Autodesk Inventor part; units mm, degrees
(part 3 of 3)
ref_plane "to_Bolt_1_434_YZ" through (140.9639, 0, 300) normal (1, 0, 0) x (0, 0, -1)
ref_plane "to_Bolt_1_434_ZX" through (140.9639, 0, 300) normal (0, 0, -1) x (0, 1, 0)
ref_plane "to_Bolt_1_435_XY" through (143.3735, 0, 300) normal (0, 1, 0) x (1, 0, 0)
ref_plane "to_Bolt_1_435_YZ" through (143.3735, 0, 300) normal (1, 0, 0) x (0, 0, -1)
ref_plane "to_Bolt_1_435_ZX" through (143.3735, 0, 300) normal (0, 0, -1) x (0, 1, 0)
ref_plane "to_Bolt_1_436_XY" through (145.7831, 0, 300) normal (0, 1, 0) x (1, 0, 0)
ref_plane "to_Bolt_1_436_YZ" through (145.7831, 0, 300) normal (1, 0, 0) x (0, 0, -1)
ref_plane "to_Bolt_1_436_ZX" through (145.7831, 0, 300) normal (0, 0, -1) x (0, 1, 0)
ref_plane "to_Bolt_1_437_XY" through (148.1928, 0, 300) normal (0, 1, 0) x (1, 0, 0)
ref_plane "to_Bolt_1_437_YZ" through (148.1928, 0, 300) normal (1, 0, 0) x (0, 0, -1)
ref_plane "to_Bolt_1_437_ZX" through (148.1928, 0, 300) normal (0, 0, -1) x (0, 1, 0)
ref_plane "to_Bolt_1_438_XY" through (150.6024, 0, 300) normal (0, 1, 0) x (1, 0, 0)
ref_plane "to_Bolt_1_438_YZ" through (150.6024, 0, 300) normal (1, 0, 0) x (0, 0, -1)
ref_plane "to_Bolt_1_438_ZX" through (150.6024, 0, 300) normal (0, 0, -1) x (0, 1, 0)
ref_plane "to_Bolt_1_439_XY" through (153.012, 0, 300) normal (0, 1, 0) x (1, 0, 0)
ref_plane "to_Bolt_1_439_YZ" through (153.012, 0, 300) normal (1, 0, 0) x (0, 0, -1)
ref_plane "to_Bolt_1_439_ZX" through (153.012, 0, 300) normal (0, 0, -1) x (0, 1, 0)
ref_plane "to_Bolt_1_44_XY" through (-196.3855, 0, -300) normal (0, 1, 0) x (1, 0, 0)
ref_plane "to_Bolt_1_44_YZ" through (-196.3855, 0, -300) normal (1, 0, 0) x (0, 0, -1)
ref_plane "to_Bolt_1_44_ZX" through (-196.3855, 0, -300) normal (0, 0, -1) x (0, 1, 0)
ref_plane "to_Bolt_1_440_XY" through (155.4217, 0, 300) normal (0, 1, 0) x (1, 0, 0)
ref_plane "to_Bolt_1_440_YZ" through (155.4217, 0, 300) normal (1, 0, 0) x (0, 0, -1)
ref_plane "to_Bolt_1_440_ZX" through (155.4217, 0, 300) normal (0, 0, -1) x (0, 1, 0)
ref_plane "to_Bolt_1_441_XY" through (157.8313, 0, 300) normal (0, 1, 0) x (1, 0, 0)
ref_plane "to_Bolt_1_441_YZ" through (157.8313, 0, 300) normal (1, 0, 0) x (0, 0, -1)
ref_plane "to_Bolt_1_441_ZX" through (157.8313, 0, 300) normal (0, 0, -1) x (0, 1, 0)
ref_plane "to_Bolt_1_442_XY" through (160.241, 0, 300) normal (0, 1, 0) x (1, 0, 0)
ref_plane "to_Bolt_1_442_YZ" through (160.241, 0, 300) normal (1, 0, 0) x (0, 0, -1)
ref_plane "to_Bolt_1_442_ZX" through (160.241, 0, 300) normal (0, 0, -1) x (0, 1, 0)
ref_plane "to_Bolt_1_443_XY" through (162.6506, 0, 300) normal (0, 1, 0) x (1, 0, 0)
ref_plane "to_Bolt_1_443_YZ" through (162.6506, 0, 300) normal (1, 0, 0) x (0, 0, -1)
ref_plane "to_Bolt_1_443_ZX" through (162.6506, 0, 300) normal (0, 0, -1) x (0, 1, 0)
ref_plane "to_Bolt_1_444_XY" through (165.0602, 0, 300) normal (0, 1, 0) x (1, 0, 0)
ref_plane "to_Bolt_1_444_YZ" through (165.0602, 0, 300) normal (1, 0, 0) x (0, 0, -1)
ref_plane "to_Bolt_1_444_ZX" through (165.0602, 0, 300) normal (0, 0, -1) x (0, 1, 0)
ref_plane "to_Bolt_1_445_XY" through (167.4699, 0, 300) normal (0, 1, 0) x (1, 0, 0)
ref_plane "to_Bolt_1_445_YZ" through (167.4699, 0, 300) normal (1, 0, 0) x (0, 0, -1)
ref_plane "to_Bolt_1_445_ZX" through (167.4699, 0, 300) normal (0, 0, -1) x (0, 1, 0)
ref_plane "to_Bolt_1_446_XY" through (169.8795, 0, 300) normal (0, 1, 0) x (1, 0, 0)
ref_plane "to_Bolt_1_446_YZ" through (169.8795, 0, 300) normal (1, 0, 0) x (0, 0, -1)
ref_plane "to_Bolt_1_446_ZX" through (169.8795, 0, 300) normal (0, 0, -1) x (0, 1, 0)
ref_plane "to_Bolt_1_447_XY" through (172.2892, 0, 300) normal (0, 1, 0) x (1, 0, 0)
ref_plane "to_Bolt_1_447_YZ" through (172.2892, 0, 300) normal (1, 0, 0) x (0, 0, -1)
ref_plane "to_Bolt_1_447_ZX" through (172.2892, 0, 300) normal (0, 0, -1) x (0, 1, 0)
ref_plane "to_Bolt_1_448_XY" through (174.6988, 0, 300) normal (0, 1, 0) x (1, 0, 0)
ref_plane "to_Bolt_1_448_YZ" through (174.6988, 0, 300) normal (1, 0, 0) x (0, 0, -1)
ref_plane "to_Bolt_1_448_ZX" through (174.6988, 0, 300) normal (0, 0, -1) x (0, 1, 0)
ref_plane "to_Bolt_1_449_XY" through (177.1084, 0, 300) normal (0, 1, 0) x (1, 0, 0)
ref_plane "to_Bolt_1_449_YZ" through (177.1084, 0, 300) normal (1, 0, 0) x (0, 0, -1)
ref_plane "to_Bolt_1_449_ZX" through (177.1084, 0, 300) normal (0, 0, -1) x (0, 1, 0)
ref_plane "to_Bolt_1_45_XY" through (-193.9759, 0, -300) normal (0, 1, 0) x (1, 0, 0)
ref_plane "to_Bolt_1_45_YZ" through (-193.9759, 0, -300) normal (1, 0, 0) x (0, 0, -1)
ref_plane "to_Bolt_1_45_ZX" through (-193.9759, 0, -300) normal (0, 0, -1) x (0, 1, 0)
ref_plane "to_Bolt_1_450_XY" through (179.5181, 0, 300) normal (0, 1, 0) x (1, 0, 0)
ref_plane "to_Bolt_1_450_YZ" through (179.5181, 0, 300) normal (1, 0, 0) x (0, 0, -1)
ref_plane "to_Bolt_1_450_ZX" through (179.5181, 0, 300) normal (0, 0, -1) x (0, 1, 0)
ref_plane "to_Bolt_1_451_XY" through (181.9277, 0, 300) normal (0, 1, 0) x (1, 0, 0)
ref_plane "to_Bolt_1_451_YZ" through (181.9277, 0, 300) normal (1, 0, 0) x (0, 0, -1)
ref_plane "to_Bolt_1_451_ZX" through (181.9277, 0, 300) normal (0, 0, -1) x (0, 1, 0)
ref_plane "to_Bolt_1_452_XY" through (184.3373, 0, 300) normal (0, 1, 0) x (1, 0, 0)
ref_plane "to_Bolt_1_452_YZ" through (184.3373, 0, 300) normal (1, 0, 0) x (0, 0, -1)
ref_plane "to_Bolt_1_452_ZX" through (184.3373, 0, 300) normal (0, 0, -1) x (0, 1, 0)
ref_plane "to_Bolt_1_453_XY" through (186.747, 0, 300) normal (0, 1, 0) x (1, 0, 0)
ref_plane "to_Bolt_1_453_YZ" through (186.747, 0, 300) normal (1, 0, 0) x (0, 0, -1)
ref_plane "to_Bolt_1_453_ZX" through (186.747, 0, 300) normal (0, 0, -1) x (0, 1, 0)
ref_plane "to_Bolt_1_454_XY" through (189.1566, 0, 300) normal (0, 1, 0) x (1, 0, 0)
ref_plane "to_Bolt_1_454_YZ" through (189.1566, 0, 300) normal (1, 0, 0) x (0, 0, -1)
ref_plane "to_Bolt_1_454_ZX" through (189.1566, 0, 300) normal (0, 0, -1) x (0, 1, 0)
ref_plane "to_Bolt_1_455_XY" through (191.5663, 0, 300) normal (0, 1, 0) x (1, 0, 0)
ref_plane "to_Bolt_1_455_YZ" through (191.5663, 0, 300) normal (1, 0, 0) x (0, 0, -1)
ref_plane "to_Bolt_1_455_ZX" through (191.5663, 0, 300) normal (0, 0, -1) x (0, 1, 0)
ref_plane "to_Bolt_1_456_XY" through (193.9759, 0, 300) normal (0, 1, 0) x (1, 0, 0)
ref_plane "to_Bolt_1_456_YZ" through (193.9759, 0, 300) normal (1, 0, 0) x (0, 0, -1)
ref_plane "to_Bolt_1_456_ZX" through (193.9759, 0, 300) normal (0, 0, -1) x (0, 1, 0)
ref_plane "to_Bolt_1_457_XY" through (196.3855, 0, 300) normal (0, 1, 0) x (1, 0, 0)
ref_plane "to_Bolt_1_457_YZ" through (196.3855, 0, 300) normal (1, 0, 0) x (0, 0, -1)
ref_plane "to_Bolt_1_457_ZX" through (196.3855, 0, 300) normal (0, 0, -1) x (0, 1, 0)
ref_plane "to_Bolt_1_458_XY" through (198.7952, 0, 300) normal (0, 1, 0) x (1, 0, 0)
ref_plane "to_Bolt_1_458_YZ" through (198.7952, 0, 300) normal (1, 0, 0) x (0, 0, -1)
ref_plane "to_Bolt_1_458_ZX" through (198.7952, 0, 300) normal (0, 0, -1) x (0, 1, 0)
ref_plane "to_Bolt_1_459_XY" through (201.2048, 0, 300) normal (0, 1, 0) x (1, 0, 0)
ref_plane "to_Bolt_1_459_YZ" through (201.2048, 0, 300) normal (1, 0, 0) x (0, 0, -1)
ref_plane "to_Bolt_1_459_ZX" through (201.2048, 0, 300) normal (0, 0, -1) x (0, 1, 0)
ref_plane "to_Bolt_1_46_XY" through (-191.5663, 0, -300) normal (0, 1, 0) x (1, 0, 0)
ref_plane "to_Bolt_1_46_YZ" through (-191.5663, 0, -300) normal (1, 0, 0) x (0, 0, -1)
ref_plane "to_Bolt_1_46_ZX" through (-191.5663, 0, -300) normal (0, 0, -1) x (0, 1, 0)
ref_plane "to_Bolt_1_460_XY" through (203.6145, 0, 300) normal (0, 1, 0) x (1, 0, 0)
ref_plane "to_Bolt_1_460_YZ" through (203.6145, 0, 300) normal (1, 0, 0) x (0, 0, -1)
ref_plane "to_Bolt_1_460_ZX" through (203.6145, 0, 300) normal (0, 0, -1) x (0, 1, 0)
ref_plane "to_Bolt_1_461_XY" through (206.0241, 0, 300) normal (0, 1, 0) x (1, 0, 0)
ref_plane "to_Bolt_1_461_YZ" through (206.0241, 0, 300) normal (1, 0, 0) x (0, 0, -1)
ref_plane "to_Bolt_1_461_ZX" through (206.0241, 0, 300) normal (0, 0, -1) x (0, 1, 0)
ref_plane "to_Bolt_1_462_XY" through (208.4337, 0, 300) normal (0, 1, 0) x (1, 0, 0)
ref_plane "to_Bolt_1_462_YZ" through (208.4337, 0, 300) normal (1, 0, 0) x (0, 0, -1)
ref_plane "to_Bolt_1_462_ZX" through (208.4337, 0, 300) normal (0, 0, -1) x (0, 1, 0)
ref_plane "to_Bolt_1_463_XY" through (210.8434, 0, 300) normal (0, 1, 0) x (1, 0, 0)
ref_plane "to_Bolt_1_463_YZ" through (210.8434, 0, 300) normal (1, 0, 0) x (0, 0, -1)
ref_plane "to_Bolt_1_463_ZX" through (210.8434, 0, 300) normal (0, 0, -1) x (0, 1, 0)
ref_plane "to_Bolt_1_464_XY" through (213.253, 0, 300) normal (0, 1, 0) x (1, 0, 0)
ref_plane "to_Bolt_1_464_YZ" through (213.253, 0, 300) normal (1, 0, 0) x (0, 0, -1)
ref_plane "to_Bolt_1_464_ZX" through (213.253, 0, 300) normal (0, 0, -1) x (0, 1, 0)
ref_plane "to_Bolt_1_465_XY" through (215.6627, 0, 300) normal (0, 1, 0) x (1, 0, 0)
ref_plane "to_Bolt_1_465_YZ" through (215.6627, 0, 300) normal (1, 0, 0) x (0, 0, -1)
ref_plane "to_Bolt_1_465_ZX" through (215.6627, 0, 300) normal (0, 0, -1) x (0, 1, 0)
ref_plane "to_Bolt_1_466_XY" through (218.0723, 0, 300) normal (0, 1, 0) x (1, 0, 0)
ref_plane "to_Bolt_1_466_YZ" through (218.0723, 0, 300) normal (1, 0, 0) x (0, 0, -1)
ref_plane "to_Bolt_1_466_ZX" through (218.0723, 0, 300) normal (0, 0, -1) x (0, 1, 0)
ref_plane "to_Bolt_1_467_XY" through (220.4819, 0, 300) normal (0, 1, 0) x (1, 0, 0)
ref_plane "to_Bolt_1_467_YZ" through (220.4819, 0, 300) normal (1, 0, 0) x (0, 0, -1)
ref_plane "to_Bolt_1_467_ZX" through (220.4819, 0, 300) normal (0, 0, -1) x (0, 1, 0)
ref_plane "to_Bolt_1_468_XY" through (222.8916, 0, 300) normal (0, 1, 0) x (1, 0, 0)
ref_plane "to_Bolt_1_468_YZ" through (222.8916, 0, 300) normal (1, 0, 0) x (0, 0, -1)
ref_plane "to_Bolt_1_468_ZX" through (222.8916, 0, 300) normal (0, 0, -1) x (0, 1, 0)
ref_plane "to_Bolt_1_469_XY" through (225.3012, 0, 300) normal (0, 1, 0) x (1, 0, 0)
ref_plane "to_Bolt_1_469_YZ" through (225.3012, 0, 300) normal (1, 0, 0) x (0, 0, -1)
ref_plane "to_Bolt_1_469_ZX" through (225.3012, 0, 300) normal (0, 0, -1) x (0, 1, 0)
ref_plane "to_Bolt_1_47_XY" through (-189.1566, 0, -300) normal (0, 1, 0) x (1, 0, 0)
ref_plane "to_Bolt_1_47_YZ" through (-189.1566, 0, -300) normal (1, 0, 0) x (0, 0, -1)
ref_plane "to_Bolt_1_47_ZX" through (-189.1566, 0, -300) normal (0, 0, -1) x (0, 1, 0)
ref_plane "to_Bolt_1_470_XY" through (227.7108, 0, 300) normal (0, 1, 0) x (1, 0, 0)
ref_plane "to_Bolt_1_470_YZ" through (227.7108, 0, 300) normal (1, 0, 0) x (0, 0, -1)
ref_plane "to_Bolt_1_470_ZX" through (227.7108, 0, 300) normal (0, 0, -1) x (0, 1, 0)
ref_plane "to_Bolt_1_471_XY" through (230.1205, 0, 300) normal (0, 1, 0) x (1, 0, 0)
ref_plane "to_Bolt_1_471_YZ" through (230.1205, 0, 300) normal (1, 0, 0) x (0, 0, -1)
ref_plane "to_Bolt_1_471_ZX" through (230.1205, 0, 300) normal (0, 0, -1) x (0, 1, 0)
ref_plane "to_Bolt_1_472_XY" through (232.5301, 0, 300) normal (0, 1, 0) x (1, 0, 0)
ref_plane "to_Bolt_1_472_YZ" through (232.5301, 0, 300) normal (1, 0, 0) x (0, 0, -1)
ref_plane "to_Bolt_1_472_ZX" through (232.5301, 0, 300) normal (0, 0, -1) x (0, 1, 0)
ref_plane "to_Bolt_1_473_XY" through (234.9398, 0, 300) normal (0, 1, 0) x (1, 0, 0)
ref_plane "to_Bolt_1_473_YZ" through (234.9398, 0, 300) normal (1, 0, 0) x (0, 0, -1)
ref_plane "to_Bolt_1_473_ZX" through (234.9398, 0, 300) normal (0, 0, -1) x (0, 1, 0)
ref_plane "to_Bolt_1_474_XY" through (237.3494, 0, 300) normal (0, 1, 0) x (1, 0, 0)
ref_plane "to_Bolt_1_474_YZ" through (237.3494, 0, 300) normal (1, 0, 0) x (0, 0, -1)
ref_plane "to_Bolt_1_474_ZX" through (237.3494, 0, 300) normal (0, 0, -1) x (0, 1, 0)
ref_plane "to_Bolt_1_475_XY" through (239.759, 0, 300) normal (0, 1, 0) x (1, 0, 0)
ref_plane "to_Bolt_1_475_YZ" through (239.759, 0, 300) normal (1, 0, 0) x (0, 0, -1)
ref_plane "to_Bolt_1_475_ZX" through (239.759, 0, 300) normal (0, 0, -1) x (0, 1, 0)
ref_plane "to_Bolt_1_476_XY" through (242.1687, 0, 300) normal (0, 1, 0) x (1, 0, 0)
ref_plane "to_Bolt_1_476_YZ" through (242.1687, 0, 300) normal (1, 0, 0) x (0, 0, -1)
ref_plane "to_Bolt_1_476_ZX" through (242.1687, 0, 300) normal (0, 0, -1) x (0, 1, 0)
ref_plane "to_Bolt_1_477_XY" through (244.5783, 0, 300) normal (0, 1, 0) x (1, 0, 0)
ref_plane "to_Bolt_1_477_YZ" through (244.5783, 0, 300) normal (1, 0, 0) x (0, 0, -1)
ref_plane "to_Bolt_1_477_ZX" through (244.5783, 0, 300) normal (0, 0, -1) x (0, 1, 0)
ref_plane "to_Bolt_1_478_XY" through (246.988, 0, 300) normal (0, 1, 0) x (1, 0, 0)
ref_plane "to_Bolt_1_478_YZ" through (246.988, 0, 300) normal (1, 0, 0) x (0, 0, -1)
ref_plane "to_Bolt_1_478_ZX" through (246.988, 0, 300) normal (0, 0, -1) x (0, 1, 0)
ref_plane "to_Bolt_1_479_XY" through (249.3976, 0, 300) normal (0, 1, 0) x (1, 0, 0)
ref_plane "to_Bolt_1_479_YZ" through (249.3976, 0, 300) normal (1, 0, 0) x (0, 0, -1)
ref_plane "to_Bolt_1_479_ZX" through (249.3976, 0, 300) normal (0, 0, -1) x (0, 1, 0)
ref_plane "to_Bolt_1_48_XY" through (-186.747, 0, -300) normal (0, 1, 0) x (1, 0, 0)
ref_plane "to_Bolt_1_48_YZ" through (-186.747, 0, -300) normal (1, 0, 0) x (0, 0, -1)
ref_plane "to_Bolt_1_48_ZX" through (-186.747, 0, -300) normal (0, 0, -1) x (0, 1, 0)
ref_plane "to_Bolt_1_480_XY" through (251.8072, 0, 300) normal (0, 1, 0) x (1, 0, 0)
ref_plane "to_Bolt_1_480_YZ" through (251.8072, 0, 300) normal (1, 0, 0) x (0, 0, -1)
ref_plane "to_Bolt_1_480_ZX" through (251.8072, 0, 300) normal (0, 0, -1) x (0, 1, 0)
ref_plane "to_Bolt_1_481_XY" through (254.2169, 0, 300) normal (0, 1, 0) x (1, 0, 0)
ref_plane "to_Bolt_1_481_YZ" through (254.2169, 0, 300) normal (1, 0, 0) x (0, 0, -1)
ref_plane "to_Bolt_1_481_ZX" through (254.2169, 0, 300) normal (0, 0, -1) x (0, 1, 0)
ref_plane "to_Bolt_1_482_XY" through (256.6265, 0, 300) normal (0, 1, 0) x (1, 0, 0)
ref_plane "to_Bolt_1_482_YZ" through (256.6265, 0, 300) normal (1, 0, 0) x (0, 0, -1)
ref_plane "to_Bolt_1_482_ZX" through (256.6265, 0, 300) normal (0, 0, -1) x (0, 1, 0)
ref_plane "to_Bolt_1_483_XY" through (259.0361, 0, 300) normal (0, 1, 0) x (1, 0, 0)
ref_plane "to_Bolt_1_483_YZ" through (259.0361, 0, 300) normal (1, 0, 0) x (0, 0, -1)
ref_plane "to_Bolt_1_483_ZX" through (259.0361, 0, 300) normal (0, 0, -1) x (0, 1, 0)
ref_plane "to_Bolt_1_484_XY" through (261.4458, 0, 300) normal (0, 1, 0) x (1, 0, 0)
ref_plane "to_Bolt_1_484_YZ" through (261.4458, 0, 300) normal (1, 0, 0) x (0, 0, -1)
ref_plane "to_Bolt_1_484_ZX" through (261.4458, 0, 300) normal (0, 0, -1) x (0, 1, 0)
ref_plane "to_Bolt_1_485_XY" through (263.8554, 0, 300) normal (0, 1, 0) x (1, 0, 0)
ref_plane "to_Bolt_1_485_YZ" through (263.8554, 0, 300) normal (1, 0, 0) x (0, 0, -1)
ref_plane "to_Bolt_1_485_ZX" through (263.8554, 0, 300) normal (0, 0, -1) x (0, 1, 0)
ref_plane "to_Bolt_1_486_XY" through (266.2651, 0, 300) normal (0, 1, 0) x (1, 0, 0)
ref_plane "to_Bolt_1_486_YZ" through (266.2651, 0, 300) normal (1, 0, 0) x (0, 0, -1)
ref_plane "to_Bolt_1_486_ZX" through (266.2651, 0, 300) normal (0, 0, -1) x (0, 1, 0)
ref_plane "to_Bolt_1_487_XY" through (268.6747, 0, 300) normal (0, 1, 0) x (1, 0, 0)
ref_plane "to_Bolt_1_487_YZ" through (268.6747, 0, 300) normal (1, 0, 0) x (0, 0, -1)
ref_plane "to_Bolt_1_487_ZX" through (268.6747, 0, 300) normal (0, 0, -1) x (0, 1, 0)
ref_plane "to_Bolt_1_488_XY" through (271.0843, 0, 300) normal (0, 1, 0) x (1, 0, 0)
ref_plane "to_Bolt_1_488_YZ" through (271.0843, 0, 300) normal (1, 0, 0) x (0, 0, -1)
ref_plane "to_Bolt_1_488_ZX" through (271.0843, 0, 300) normal (0, 0, -1) x (0, 1, 0)
ref_plane "to_Bolt_1_489_XY" through (273.494, 0, 300) normal (0, 1, 0) x (1, 0, 0)
ref_plane "to_Bolt_1_489_YZ" through (273.494, 0, 300) normal (1, 0, 0) x (0, 0, -1)
ref_plane "to_Bolt_1_489_ZX" through (273.494, 0, 300) normal (0, 0, -1) x (0, 1, 0)
ref_plane "to_Bolt_1_49_XY" through (-184.3373, 0, -300) normal (0, 1, 0) x (1, 0, 0)
ref_plane "to_Bolt_1_49_YZ" through (-184.3373, 0, -300) normal (1, 0, 0) x (0, 0, -1)
ref_plane "to_Bolt_1_49_ZX" through (-184.3373, 0, -300) normal (0, 0, -1) x (0, 1, 0)
ref_plane "to_Bolt_1_490_XY" through (275.9036, 0, 300) normal (0, 1, 0) x (1, 0, 0)
ref_plane "to_Bolt_1_490_YZ" through (275.9036, 0, 300) normal (1, 0, 0) x (0, 0, -1)
ref_plane "to_Bolt_1_490_ZX" through (275.9036, 0, 300) normal (0, 0, -1) x (0, 1, 0)
ref_plane "to_Bolt_1_491_XY" through (278.3133, 0, 300) normal (0, 1, 0) x (1, 0, 0)
ref_plane "to_Bolt_1_491_YZ" through (278.3133, 0, 300) normal (1, 0, 0) x (0, 0, -1)
ref_plane "to_Bolt_1_491_ZX" through (278.3133, 0, 300) normal (0, 0, -1) x (0, 1, 0)
ref_plane "to_Bolt_1_492_XY" through (280.7229, 0, 300) normal (0, 1, 0) x (1, 0, 0)
ref_plane "to_Bolt_1_492_YZ" through (280.7229, 0, 300) normal (1, 0, 0) x (0, 0, -1)
ref_plane "to_Bolt_1_492_ZX" through (280.7229, 0, 300) normal (0, 0, -1) x (0, 1, 0)
ref_plane "to_Bolt_1_493_XY" through (283.1325, 0, 300) normal (0, 1, 0) x (1, 0, 0)
ref_plane "to_Bolt_1_493_YZ" through (283.1325, 0, 300) normal (1, 0, 0) x (0, 0, -1)
ref_plane "to_Bolt_1_493_ZX" through (283.1325, 0, 300) normal (0, 0, -1) x (0, 1, 0)
ref_plane "to_Bolt_1_494_XY" through (285.5422, 0, 300) normal (0, 1, 0) x (1, 0, 0)
ref_plane "to_Bolt_1_494_YZ" through (285.5422, 0, 300) normal (1, 0, 0) x (0, 0, -1)
ref_plane "to_Bolt_1_494_ZX" through (285.5422, 0, 300) normal (0, 0, -1) x (0, 1, 0)
ref_plane "to_Bolt_1_495_XY" through (287.9518, 0, 300) normal (0, 1, 0) x (1, 0, 0)
ref_plane "to_Bolt_1_495_YZ" through (287.9518, 0, 300) normal (1, 0, 0) x (0, 0, -1)
ref_plane "to_Bolt_1_495_ZX" through (287.9518, 0, 300) normal (0, 0, -1) x (0, 1, 0)
ref_plane "to_Bolt_1_496_XY" through (290.3614, 0, 300) normal (0, 1, 0) x (1, 0, 0)
ref_plane "to_Bolt_1_496_YZ" through (290.3614, 0, 300) normal (1, 0, 0) x (0, 0, -1)
ref_plane "to_Bolt_1_496_ZX" through (290.3614, 0, 300) normal (0, 0, -1) x (0, 1, 0)
ref_plane "to_Bolt_1_497_XY" through (292.7711, 0, 300) normal (0, 1, 0) x (1, 0, 0)
ref_plane "to_Bolt_1_497_YZ" through (292.7711, 0, 300) normal (1, 0, 0) x (0, 0, -1)
ref_plane "to_Bolt_1_497_ZX" through (292.7711, 0, 300) normal (0, 0, -1) x (0, 1, 0)
ref_plane "to_Bolt_1_498_XY" through (295.1807, 0, 300) normal (0, 1, 0) x (1, 0, 0)
ref_plane "to_Bolt_1_498_YZ" through (295.1807, 0, 300) normal (1, 0, 0) x (0, 0, -1)
ref_plane "to_Bolt_1_498_ZX" through (295.1807, 0, 300) normal (0, 0, -1) x (0, 1, 0)
ref_plane "to_Bolt_1_499_XY" through (297.5904, 0, 300) normal (0, 1, 0) x (1, 0, 0)
ref_plane "to_Bolt_1_499_YZ" through (297.5904, 0, 300) normal (1, 0, 0) x (0, 0, -1)
ref_plane "to_Bolt_1_499_ZX" through (297.5904, 0, 300) normal (0, 0, -1) x (0, 1, 0)
ref_plane "to_Bolt_1_5_XY" through (-290.3614, 0, -300) normal (0, 1, 0) x (1, 0, 0)
ref_plane "to_Bolt_1_5_YZ" through (-290.3614, 0, -300) normal (1, 0, 0) x (0, 0, -1)
ref_plane "to_Bolt_1_5_ZX" through (-290.3614, 0, -300) normal (0, 0, -1) x (0, 1, 0)
ref_plane "to_Bolt_1_50_XY" through (-181.9277, 0, -300) normal (0, 1, 0) x (1, 0, 0)
ref_plane "to_Bolt_1_50_YZ" through (-181.9277, 0, -300) normal (1, 0, 0) x (0, 0, -1)
ref_plane "to_Bolt_1_50_ZX" through (-181.9277, 0, -300) normal (0, 0, -1) x (0, 1, 0)
ref_plane "to_Bolt_1_500_XY" through (300, 0, 300) normal (0, 1, 0) x (1, 0, 0)
ref_plane "to_Bolt_1_500_YZ" through (300, 0, 300) normal (1, 0, 0) x (0, 0, -1)
ref_plane "to_Bolt_1_500_ZX" through (300, 0, 300) normal (0, 0, -1) x (0, 1, 0)
ref_plane "to_Bolt_1_51_XY" through (-179.5181, 0, -300) normal (0, 1, 0) x (1, 0, 0)
ref_plane "to_Bolt_1_51_YZ" through (-179.5181, 0, -300) normal (1, 0, 0) x (0, 0, -1)
ref_plane "to_Bolt_1_51_ZX" through (-179.5181, 0, -300) normal (0, 0, -1) x (0, 1, 0)
ref_plane "to_Bolt_1_52_XY" through (-177.1084, 0, -300) normal (0, 1, 0) x (1, 0, 0)
ref_plane "to_Bolt_1_52_YZ" through (-177.1084, 0, -300) normal (1, 0, 0) x (0, 0, -1)
ref_plane "to_Bolt_1_52_ZX" through (-177.1084, 0, -300) normal (0, 0, -1) x (0, 1, 0)
ref_plane "to_Bolt_1_53_XY" through (-174.6988, 0, -300) normal (0, 1, 0) x (1, 0, 0)
ref_plane "to_Bolt_1_53_YZ" through (-174.6988, 0, -300) normal (1, 0, 0) x (0, 0, -1)
ref_plane "to_Bolt_1_53_ZX" through (-174.6988, 0, -300) normal (0, 0, -1) x (0, 1, 0)
ref_plane "to_Bolt_1_54_XY" through (-172.2892, 0, -300) normal (0, 1, 0) x (1, 0, 0)
ref_plane "to_Bolt_1_54_YZ" through (-172.2892, 0, -300) normal (1, 0, 0) x (0, 0, -1)
ref_plane "to_Bolt_1_54_ZX" through (-172.2892, 0, -300) normal (0, 0, -1) x (0, 1, 0)
ref_plane "to_Bolt_1_55_XY" through (-169.8795, 0, -300) normal (0, 1, 0) x (1, 0, 0)
ref_plane "to_Bolt_1_55_YZ" through (-169.8795, 0, -300) normal (1, 0, 0) x (0, 0, -1)
ref_plane "to_Bolt_1_55_ZX" through (-169.8795, 0, -300) normal (0, 0, -1) x (0, 1, 0)
ref_plane "to_Bolt_1_56_XY" through (-167.4699, 0, -300) normal (0, 1, 0) x (1, 0, 0)
ref_plane "to_Bolt_1_56_YZ" through (-167.4699, 0, -300) normal (1, 0, 0) x (0, 0, -1)
ref_plane "to_Bolt_1_56_ZX" through (-167.4699, 0, -300) normal (0, 0, -1) x (0, 1, 0)
ref_plane "to_Bolt_1_57_XY" through (-165.0602, 0, -300) normal (0, 1, 0) x (1, 0, 0)
ref_plane "to_Bolt_1_57_YZ" through (-165.0602, 0, -300) normal (1, 0, 0) x (0, 0, -1)
ref_plane "to_Bolt_1_57_ZX" through (-165.0602, 0, -300) normal (0, 0, -1) x (0, 1, 0)
ref_plane "to_Bolt_1_58_XY" through (-162.6506, 0, -300) normal (0, 1, 0) x (1, 0, 0)
ref_plane "to_Bolt_1_58_YZ" through (-162.6506, 0, -300) normal (1, 0, 0) x (0, 0, -1)
ref_plane "to_Bolt_1_58_ZX" through (-162.6506, 0, -300) normal (0, 0, -1) x (0, 1, 0)
ref_plane "to_Bolt_1_59_XY" through (-160.241, 0, -300) normal (0, 1, 0) x (1, 0, 0)
ref_plane "to_Bolt_1_59_YZ" through (-160.241, 0, -300) normal (1, 0, 0) x (0, 0, -1)
ref_plane "to_Bolt_1_59_ZX" through (-160.241, 0, -300) normal (0, 0, -1) x (0, 1, 0)
ref_plane "to_Bolt_1_6_XY" through (-287.9518, 0, -300) normal (0, 1, 0) x (1, 0, 0)
ref_plane "to_Bolt_1_6_YZ" through (-287.9518, 0, -300) normal (1, 0, 0) x (0, 0, -1)
ref_plane "to_Bolt_1_6_ZX" through (-287.9518, 0, -300) normal (0, 0, -1) x (0, 1, 0)
ref_plane "to_Bolt_1_60_XY" through (-157.8313, 0, -300) normal (0, 1, 0) x (1, 0, 0)
ref_plane "to_Bolt_1_60_YZ" through (-157.8313, 0, -300) normal (1, 0, 0) x (0, 0, -1)
ref_plane "to_Bolt_1_60_ZX" through (-157.8313, 0, -300) normal (0, 0, -1) x (0, 1, 0)
ref_plane "to_Bolt_1_61_XY" through (-155.4217, 0, -300) normal (0, 1, 0) x (1, 0, 0)
ref_plane "to_Bolt_1_61_YZ" through (-155.4217, 0, -300) normal (1, 0, 0) x (0, 0, -1)
ref_plane "to_Bolt_1_61_ZX" through (-155.4217, 0, -300) normal (0, 0, -1) x (0, 1, 0)
ref_plane "to_Bolt_1_62_XY" through (-153.012, 0, -300) normal (0, 1, 0) x (1, 0, 0)
ref_plane "to_Bolt_1_62_YZ" through (-153.012, 0, -300) normal (1, 0, 0) x (0, 0, -1)
ref_plane "to_Bolt_1_62_ZX" through (-153.012, 0, -300) normal (0, 0, -1) x (0, 1, 0)
ref_plane "to_Bolt_1_63_XY" through (-150.6024, 0, -300) normal (0, 1, 0) x (1, 0, 0)
ref_plane "to_Bolt_1_63_YZ" through (-150.6024, 0, -300) normal (1, 0, 0) x (0, 0, -1)
ref_plane "to_Bolt_1_63_ZX" through (-150.6024, 0, -300) normal (0, 0, -1) x (0, 1, 0)
ref_plane "to_Bolt_1_64_XY" through (-148.1928, 0, -300) normal (0, 1, 0) x (1, 0, 0)
ref_plane "to_Bolt_1_64_YZ" through (-148.1928, 0, -300) normal (1, 0, 0) x (0, 0, -1)
ref_plane "to_Bolt_1_64_ZX" through (-148.1928, 0, -300) normal (0, 0, -1) x (0, 1, 0)
ref_plane "to_Bolt_1_65_XY" through (-145.7831, 0, -300) normal (0, 1, 0) x (1, 0, 0)
ref_plane "to_Bolt_1_65_YZ" through (-145.7831, 0, -300) normal (1, 0, 0) x (0, 0, -1)
ref_plane "to_Bolt_1_65_ZX" through (-145.7831, 0, -300) normal (0, 0, -1) x (0, 1, 0)
ref_plane "to_Bolt_1_66_XY" through (-143.3735, 0, -300) normal (0, 1, 0) x (1, 0, 0)
ref_plane "to_Bolt_1_66_YZ" through (-143.3735, 0, -300) normal (1, 0, 0) x (0, 0, -1)
ref_plane "to_Bolt_1_66_ZX" through (-143.3735, 0, -300) normal (0, 0, -1) x (0, 1, 0)
ref_plane "to_Bolt_1_67_XY" through (-140.9639, 0, -300) normal (0, 1, 0) x (1, 0, 0)
ref_plane "to_Bolt_1_67_YZ" through (-140.9639, 0, -300) normal (1, 0, 0) x (0, 0, -1)
ref_plane "to_Bolt_1_67_ZX" through (-140.9639, 0, -300) normal (0, 0, -1) x (0, 1, 0)
ref_plane "to_Bolt_1_68_XY" through (-138.5542, 0, -300) normal (0, 1, 0) x (1, 0, 0)
ref_plane "to_Bolt_1_68_YZ" through (-138.5542, 0, -300) normal (1, 0, 0) x (0, 0, -1)
ref_plane "to_Bolt_1_68_ZX" through (-138.5542, 0, -300) normal (0, 0, -1) x (0, 1, 0)
ref_plane "to_Bolt_1_69_XY" through (-136.1446, 0, -300) normal (0, 1, 0) x (1, 0, 0)
ref_plane "to_Bolt_1_69_YZ" through (-136.1446, 0, -300) normal (1, 0, 0) x (0, 0, -1)
ref_plane "to_Bolt_1_69_ZX" through (-136.1446, 0, -300) normal (0, 0, -1) x (0, 1, 0)
ref_plane "to_Bolt_1_7_XY" through (-285.5422, 0, -300) normal (0, 1, 0) x (1, 0, 0)
ref_plane "to_Bolt_1_7_YZ" through (-285.5422, 0, -300) normal (1, 0, 0) x (0, 0, -1)
ref_plane "to_Bolt_1_7_ZX" through (-285.5422, 0, -300) normal (0, 0, -1) x (0, 1, 0)
ref_plane "to_Bolt_1_70_XY" through (-133.7349, 0, -300) normal (0, 1, 0) x (1, 0, 0)
ref_plane "to_Bolt_1_70_YZ" through (-133.7349, 0, -300) normal (1, 0, 0) x (0, 0, -1)
ref_plane "to_Bolt_1_70_ZX" through (-133.7349, 0, -300) normal (0, 0, -1) x (0, 1, 0)
ref_plane "to_Bolt_1_71_XY" through (-131.3253, 0, -300) normal (0, 1, 0) x (1, 0, 0)
ref_plane "to_Bolt_1_71_YZ" through (-131.3253, 0, -300) normal (1, 0, 0) x (0, 0, -1)
ref_plane "to_Bolt_1_71_ZX" through (-131.3253, 0, -300) normal (0, 0, -1) x (0, 1, 0)
ref_plane "to_Bolt_1_72_XY" through (-128.9157, 0, -300) normal (0, 1, 0) x (1, 0, 0)
ref_plane "to_Bolt_1_72_YZ" through (-128.9157, 0, -300) normal (1, 0, 0) x (0, 0, -1)
ref_plane "to_Bolt_1_72_ZX" through (-128.9157, 0, -300) normal (0, 0, -1) x (0, 1, 0)
ref_plane "to_Bolt_1_73_XY" through (-126.506, 0, -300) normal (0, 1, 0) x (1, 0, 0)
ref_plane "to_Bolt_1_73_YZ" through (-126.506, 0, -300) normal (1, 0, 0) x (0, 0, -1)
ref_plane "to_Bolt_1_73_ZX" through (-126.506, 0, -300) normal (0, 0, -1) x (0, 1, 0)
ref_plane "to_Bolt_1_74_XY" through (-124.0964, 0, -300) normal (0, 1, 0) x (1, 0, 0)
ref_plane "to_Bolt_1_74_YZ" through (-124.0964, 0, -300) normal (1, 0, 0) x (0, 0, -1)
ref_plane "to_Bolt_1_74_ZX" through (-124.0964, 0, -300) normal (0, 0, -1) x (0, 1, 0)
ref_plane "to_Bolt_1_75_XY" through (-121.6867, 0, -300) normal (0, 1, 0) x (1, 0, 0)
ref_plane "to_Bolt_1_75_YZ" through (-121.6867, 0, -300) normal (1, 0, 0) x (0, 0, -1)
ref_plane "to_Bolt_1_75_ZX" through (-121.6867, 0, -300) normal (0, 0, -1) x (0, 1, 0)
ref_plane "to_Bolt_1_76_XY" through (-119.2771, 0, -300) normal (0, 1, 0) x (1, 0, 0)
ref_plane "to_Bolt_1_76_YZ" through (-119.2771, 0, -300) normal (1, 0, 0) x (0, 0, -1)
ref_plane "to_Bolt_1_76_ZX" through (-119.2771, 0, -300) normal (0, 0, -1) x (0, 1, 0)
ref_plane "to_Bolt_1_77_XY" through (-116.8675, 0, -300) normal (0, 1, 0) x (1, 0, 0)
ref_plane "to_Bolt_1_77_YZ" through (-116.8675, 0, -300) normal (1, 0, 0) x (0, 0, -1)
ref_plane "to_Bolt_1_77_ZX" through (-116.8675, 0, -300) normal (0, 0, -1) x (0, 1, 0)
ref_plane "to_Bolt_1_78_XY" through (-114.4578, 0, -300) normal (0, 1, 0) x (1, 0, 0)
ref_plane "to_Bolt_1_78_YZ" through (-114.4578, 0, -300) normal (1, 0, 0) x (0, 0, -1)
ref_plane "to_Bolt_1_78_ZX" through (-114.4578, 0, -300) normal (0, 0, -1) x (0, 1, 0)
ref_plane "to_Bolt_1_79_XY" through (-112.0482, 0, -300) normal (0, 1, 0) x (1, 0, 0)
ref_plane "to_Bolt_1_79_YZ" through (-112.0482, 0, -300) normal (1, 0, 0) x (0, 0, -1)
ref_plane "to_Bolt_1_79_ZX" through (-112.0482, 0, -300) normal (0, 0, -1) x (0, 1, 0)
ref_plane "to_Bolt_1_8_XY" through (-283.1325, 0, -300) normal (0, 1, 0) x (1, 0, 0)
ref_plane "to_Bolt_1_8_YZ" through (-283.1325, 0, -300) normal (1, 0, 0) x (0, 0, -1)
ref_plane "to_Bolt_1_8_ZX" through (-283.1325, 0, -300) normal (0, 0, -1) x (0, 1, 0)
ref_plane "to_Bolt_1_80_XY" through (-109.6386, 0, -300) normal (0, 1, 0) x (1, 0, 0)
ref_plane "to_Bolt_1_80_YZ" through (-109.6386, 0, -300) normal (1, 0, 0) x (0, 0, -1)
ref_plane "to_Bolt_1_80_ZX" through (-109.6386, 0, -300) normal (0, 0, -1) x (0, 1, 0)
ref_plane "to_Bolt_1_81_XY" through (-107.2289, 0, -300) normal (0, 1, 0) x (1, 0, 0)
ref_plane "to_Bolt_1_81_YZ" through (-107.2289, 0, -300) normal (1, 0, 0) x (0, 0, -1)
ref_plane "to_Bolt_1_81_ZX" through (-107.2289, 0, -300) normal (0, 0, -1) x (0, 1, 0)
ref_plane "to_Bolt_1_82_XY" through (-104.8193, 0, -300) normal (0, 1, 0) x (1, 0, 0)
ref_plane "to_Bolt_1_82_YZ" through (-104.8193, 0, -300) normal (1, 0, 0) x (0, 0, -1)
ref_plane "to_Bolt_1_82_ZX" through (-104.8193, 0, -300) normal (0, 0, -1) x (0, 1, 0)
ref_plane "to_Bolt_1_83_XY" through (-102.4096, 0, -300) normal (0, 1, 0) x (1, 0, 0)
ref_plane "to_Bolt_1_83_YZ" through (-102.4096, 0, -300) normal (1, 0, 0) x (0, 0, -1)
ref_plane "to_Bolt_1_83_ZX" through (-102.4096, 0, -300) normal (0, 0, -1) x (0, 1, 0)
ref_plane "to_Bolt_1_84_XY" through (-100, 0, -300) normal (0, 1, 0) x (1, 0, 0)
ref_plane "to_Bolt_1_84_YZ" through (-100, 0, -300) normal (1, 0, 0) x (0, 0, -1)
ref_plane "to_Bolt_1_84_ZX" through (-100, 0, -300) normal (0, 0, -1) x (0, 1, 0)
ref_plane "to_Bolt_1_85_XY" through (-97.5904, 0, -300) normal (0, 1, 0) x (1, 0, 0)
ref_plane "to_Bolt_1_85_YZ" through (-97.5904, 0, -300) normal (1, 0, 0) x (0, 0, -1)
ref_plane "to_Bolt_1_85_ZX" through (-97.5904, 0, -300) normal (0, 0, -1) x (0, 1, 0)
ref_plane "to_Bolt_1_86_XY" through (-95.1807, 0, -300) normal (0, 1, 0) x (1, 0, 0)
ref_plane "to_Bolt_1_86_YZ" through (-95.1807, 0, -300) normal (1, 0, 0) x (0, 0, -1)
ref_plane "to_Bolt_1_86_ZX" through (-95.1807, 0, -300) normal (0, 0, -1) x (0, 1, 0)
ref_plane "to_Bolt_1_87_XY" through (-92.7711, 0, -300) normal (0, 1, 0) x (1, 0, 0)
ref_plane "to_Bolt_1_87_YZ" through (-92.7711, 0, -300) normal (1, 0, 0) x (0, 0, -1)
ref_plane "to_Bolt_1_87_ZX" through (-92.7711, 0, -300) normal (0, 0, -1) x (0, 1, 0)
ref_plane "to_Bolt_1_88_XY" through (-90.3614, 0, -300) normal (0, 1, 0) x (1, 0, 0)
ref_plane "to_Bolt_1_88_YZ" through (-90.3614, 0, -300) normal (1, 0, 0) x (0, 0, -1)
ref_plane "to_Bolt_1_88_ZX" through (-90.3614, 0, -300) normal (0, 0, -1) x (0, 1, 0)
ref_plane "to_Bolt_1_89_XY" through (-87.9518, 0, -300) normal (0, 1, 0) x (1, 0, 0)
ref_plane "to_Bolt_1_89_YZ" through (-87.9518, 0, -300) normal (1, 0, 0) x (0, 0, -1)
ref_plane "to_Bolt_1_89_ZX" through (-87.9518, 0, -300) normal (0, 0, -1) x (0, 1, 0)
ref_plane "to_Bolt_1_9_XY" through (-280.7229, 0, -300) normal (0, 1, 0) x (1, 0, 0)
ref_plane "to_Bolt_1_9_YZ" through (-280.7229, 0, -300) normal (1, 0, 0) x (0, 0, -1)
ref_plane "to_Bolt_1_9_ZX" through (-280.7229, 0, -300) normal (0, 0, -1) x (0, 1, 0)
ref_plane "to_Bolt_1_90_XY" through (-85.5422, 0, -300) normal (0, 1, 0) x (1, 0, 0)
ref_plane "to_Bolt_1_90_YZ" through (-85.5422, 0, -300) normal (1, 0, 0) x (0, 0, -1)
ref_plane "to_Bolt_1_90_ZX" through (-85.5422, 0, -300) normal (0, 0, -1) x (0, 1, 0)
ref_plane "to_Bolt_1_91_XY" through (-83.1325, 0, -300) normal (0, 1, 0) x (1, 0, 0)
ref_plane "to_Bolt_1_91_YZ" through (-83.1325, 0, -300) normal (1, 0, 0) x (0, 0, -1)
ref_plane "to_Bolt_1_91_ZX" through (-83.1325, 0, -300) normal (0, 0, -1) x (0, 1, 0)
ref_plane "to_Bolt_1_92_XY" through (-80.7229, 0, -300) normal (0, 1, 0) x (1, 0, 0)
ref_plane "to_Bolt_1_92_YZ" through (-80.7229, 0, -300) normal (1, 0, 0) x (0, 0, -1)
ref_plane "to_Bolt_1_92_ZX" through (-80.7229, 0, -300) normal (0, 0, -1) x (0, 1, 0)
ref_plane "to_Bolt_1_93_XY" through (-78.3133, 0, -300) normal (0, 1, 0) x (1, 0, 0)
ref_plane "to_Bolt_1_93_YZ" through (-78.3133, 0, -300) normal (1, 0, 0) x (0, 0, -1)
ref_plane "to_Bolt_1_93_ZX" through (-78.3133, 0, -300) normal (0, 0, -1) x (0, 1, 0)
ref_plane "to_Bolt_1_94_XY" through (-75.9036, 0, -300) normal (0, 1, 0) x (1, 0, 0)
ref_plane "to_Bolt_1_94_YZ" through (-75.9036, 0, -300) normal (1, 0, 0) x (0, 0, -1)
ref_plane "to_Bolt_1_94_ZX" through (-75.9036, 0, -300) normal (0, 0, -1) x (0, 1, 0)
ref_plane "to_Bolt_1_95_XY" through (-73.494, 0, -300) normal (0, 1, 0) x (1, 0, 0)
ref_plane "to_Bolt_1_95_YZ" through (-73.494, 0, -300) normal (1, 0, 0) x (0, 0, -1)
ref_plane "to_Bolt_1_95_ZX" through (-73.494, 0, -300) normal (0, 0, -1) x (0, 1, 0)
ref_plane "to_Bolt_1_96_XY" through (-71.0843, 0, -300) normal (0, 1, 0) x (1, 0, 0)
ref_plane "to_Bolt_1_96_YZ" through (-71.0843, 0, -300) normal (1, 0, 0) x (0, 0, -1)
ref_plane "to_Bolt_1_96_ZX" through (-71.0843, 0, -300) normal (0, 0, -1) x (0, 1, 0)
ref_plane "to_Bolt_1_97_XY" through (-68.6747, 0, -300) normal (0, 1, 0) x (1, 0, 0)
ref_plane "to_Bolt_1_97_YZ" through (-68.6747, 0, -300) normal (1, 0, 0) x (0, 0, -1)
ref_plane "to_Bolt_1_97_ZX" through (-68.6747, 0, -300) normal (0, 0, -1) x (0, 1, 0)
ref_plane "to_Bolt_1_98_XY" through (-66.2651, 0, -300) normal (0, 1, 0) x (1, 0, 0)
ref_plane "to_Bolt_1_98_YZ" through (-66.2651, 0, -300) normal (1, 0, 0) x (0, 0, -1)
ref_plane "to_Bolt_1_98_ZX" through (-66.2651, 0, -300) normal (0, 0, -1) x (0, 1, 0)
ref_plane "to_Bolt_1_99_XY" through (-63.8554, 0, -300) normal (0, 1, 0) x (1, 0, 0)
ref_plane "to_Bolt_1_99_YZ" through (-63.8554, 0, -300) normal (1, 0, 0) x (0, 0, -1)
ref_plane "to_Bolt_1_99_ZX" through (-63.8554, 0, -300) normal (0, 0, -1) x (0, 1, 0)
ref_plane "to_Bolt_2_XY" through (300, 0, -300) normal (0, 1, 0) x (1, 0, 0)
ref_plane "to_Bolt_2_YZ" through (300, 0, -300) normal (1, 0, 0) x (0, 0, -1)
ref_plane "to_Bolt_2_ZX" through (300, 0, -300) normal (0, 0, -1) x (0, 1, 0)
ref_plane "to_Bolt_3_XY" through (-300, 0, 300) normal (0, 1, 0) x (1, 0, 0)
ref_plane "to_Bolt_3_YZ" through (-300, 0, 300) normal (1, 0, 0) x (0, 0, -1)
ref_plane "to_Bolt_3_ZX" through (-300, 0, 300) normal (0, 0, -1) x (0, 1, 0)
ref_plane "to_Bolt_4_XY" through (300, 0, 300) normal (0, 1, 0) x (1, 0, 0)
ref_plane "to_Bolt_4_YZ" through (300, 0, 300) normal (1, 0, 0) x (0, 0, -1)
ref_plane "to_Bolt_4_ZX" through (300, 0, 300) normal (0, 0, -1) x (0, 1, 0)
body "Solid1"
